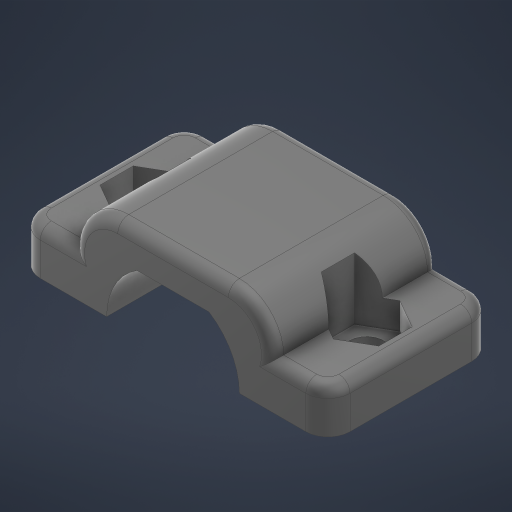
# Autodesk Inventor part: mocowanie_silnika_CPY
Saved by Autodesk Inventor 2024 (Build 280153000, 153)
## iProperties
Created: 2024-05-23
Part Number: mocowanie_silnika_CPY
Material: ABS Plastic
Document SubType Name: Modeling
Designer: Adam
Density: 1.06 g/cm^3
Appearance: Smooth - White
Author: Adam
Autodesk Inventor part; units mm, degrees
ref_plane "YZ Plane" through (0, 0, 0) normal (1, 0, 0) x (0, 1, 0)
sketch "Sketch3" plane through (0, 0, 0) normal (0, 0, 1) x (1, 0, 0)
  line L0 (2.4271, 1.3674) -> (5.6771, 1.3674)
  arc A0 (8.4273, -3.6326) -> (5.6771, 1.3674) centre (2.5072, -3.6326) ccw
  line L1 (8.4273, -3.6326) -> (8.4273, -3.6326)
  line L2 (8.4273, -3.6326) -> (16.4273, -3.6326)
  line L3 (16.4273, -3.6326) -> (16.4273, 0.3674)
  line L4 (16.4273, 0.3674) -> (11.4273, 0.3674)
  line L5 (2.4271, 4.3674) -> (7.4273, 4.3674)
  line L6 (11.4273, 0.3674) -> (11.4273, 0.3674)
  arc A1 (11.4273, 0.3674) -> (7.4273, 4.3674) centre (7.4273, 0.3674) ccw
  arc A2 (-0.8229, 1.3674) -> (-3.5732, -3.6326) centre (2.3469, -3.6326) ccw
  line L7 (-3.5732, -3.6326) -> (-3.5732, -3.6326)
  line L8 (-3.5732, -3.6326) -> (-11.5732, -3.6326)
  line L9 (-11.5732, -3.6326) -> (-11.5732, 0.3674)
  line L10 (-11.5732, 0.3674) -> (-6.5732, 0.3674)
  line L11 (-6.5732, 0.3674) -> (-6.5732, 0.3674)
  arc A3 (-2.5732, 4.3674) -> (-6.5732, 0.3674) centre (-2.5732, 0.3674) ccw
  line L12 (2.4271, 4.3674) -> (-2.5732, 4.3674)
  line L13 (2.4271, 1.3674) -> (-0.8229, 1.3674)
  point P0 (0, 0)
  point P1 (11.4273, 0.3674)
  point P2 (-6.5732, 0.3674)
  dimension "d20" = 4
  dimension "d21" = 5
  dimension "d22" = 8
  dimension "d23" = 3
  constraints: 28 end point, 8 point on circle, 4 centre point, 3 perpendicular, 2 horizontal, 2 tangent, 1 vertical, 1 other
  measures "d20" distance of L2.end L3.end
  measures "d21" distance of L3.end L6.end
  measures "d22" distance between parallel lines of L5 L2
  measures "d23" distance between parallel lines of L5 L0
extrude "Extrusion2" add sketch "Sketch3" along normal blind 15
ref_plane "Work Plane1" through (2.4271, -3.6326, 0) normal (-1, 0, 0) x (0, 0, 1)
sketch "Sketch4" plane through (-11.5732, 0.3674, 0) normal (0, 1, 0) x (1, 0, 0)
  line L0 (4, -4.495) -> (6.6024, -5.9975)
  line L1 (6.6024, -5.9975) -> (6.6024, -9.0025)
  line L2 (6.6024, -9.0025) -> (4, -10.505)
  line L3 (4, -10.505) -> (1.3976, -9.0025)
  line L4 (1.3976, -9.0025) -> (1.3976, -5.9975)
  line L5 (1.3976, -5.9975) -> (4, -4.495)
  line L6 (0, 0) -> (0, -15) projected
  line L7 (14.0003, -18) -> (14.0003, 3) projected
  line L8 (5, 0) -> (0, 0) projected
  point P0 (11.5732, 0)
  point P1 (4, -7.5)
  point P2 (4, -7.5)
  dimension "d26" = 6.01
  dimension "d27" = 4
  dimension "d39" = 7.5
  constraints: 12 end point, 1 coincident, 13 other
  measures "d26" distance of L0.start L2.end
  measures "d27" distance from line of L6 point (4, -7.5)
  measures "d39" distance from line of L8 point (4, -7.5)
extrude "Extrusion3" cut sketch "Sketch4" along normal blind 8 and the other way blind 2.4
sketch "Sketch5" plane through (-11.5732, -2.0326, 0) normal (0, 1, 0) x (1, 0, 0)
  line L0 (6.6024, -5.9975) -> (6.6024, -9.0025) projected
  line L1 (1.3976, -9.0025) -> (1.3976, -5.9975) projected
  line L2 (5, 0) -> (0, 0) projected
  point P0 (11.5732, 0)
  point P1 (4, -7.5)
  dimension "d40" = 7.5
  measures "d40" distance from line of L2 point (4, -7.5)
hole "Hole1" at (-7.5732, -2.0326, 7.5) direction (0, -1, 0) diameter 3.1 end through all
mirror "Mirror1" about plane through (2.4271, -3.6326, 0) normal (-1, 0, 0) of "Extrusion3", "Hole1"
ref_plane "Work Plane2" through (0, 0, 7.5) normal (0, 0, 1) x (1, 0, 0)
fillet "Fillet3" radius 2 4 edges at (16.4273, -1.6326, 0) (16.4273, -1.6326, 15) (-11.5732, -1.6326, 15) (-11.5732, -1.6326, 0)
fillet "Fillet4" radius 1 16 edges at (15.8415, 0.3674, 0.5858) (16.4273, 0.3674, 7.5) (15.8415, 0.3674, 14.4142) (12.9273, 0.3674, 15) (12.9273, 0.3674, 0) (2.4271, 4.3674, 0) (-5.4016, 3.1958, 0) (10.2558, 3.1958, 0) (-8.0732, 0.3674, 0) (-11.5732, 0.3674, 7.5) (-10.9874, 0.3674, 14.4142) (-8.0732, 0.3674, 15) (-10.9874, 0.3674, 0.5858) (2.4271, 4.3674, 15) (10.2558, 3.1958, 15) (-5.4016, 3.1958, 15)
body "Solid1"
